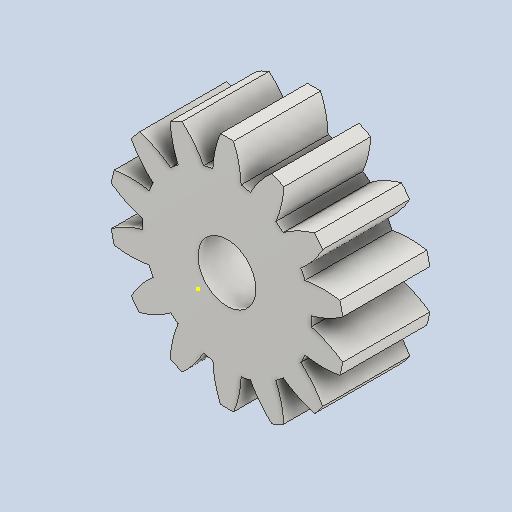
# Autodesk Inventor part: Spur Gear2
Saved by Autodesk Inventor 2022.3 (Build 263350000, 350)
## iProperties
CustomPartVersion: 1
Created: 2023-01-16
Part Number: Spur Gear2
Material: Steel
Document SubType Name: Modeling
Designer: komputer
Categories: <?xml version="1.0" encoding="UTF-16"?> <MemberInstance><Categories><FamilyTemplate><FamilyTemplateParameter ValueType="xs:double" Id="1" ObjectReferenceKey="da_z" ObjectType="kUserParameterObject"/><FamilyTemplateParameter ValueType="xs:double" Id="2" ObjectReferenceKey="da_b" ObjectType="kUserParameterObject"/><FamilyTemplateParameter ValueType="xs:double" Id="3" ObjectReferenceKey="da_beta" ObjectType="kUserParameterObject"/><FamilyTemplateParameter ValueType="xs:double" Id="4" ObjectReferenceKey="da_da" ObjectType="kUserParameterObject"/><FamilyTemplateParameter ValueType="xs:double" Id="5" ObjectReferenceKey="da_aw" ObjectType="kUserParameterObject"/><FamilyTemplateParameter ValueType="xs:string" Id="6" ObjectReferenceKey="EAIAABAAAACIAQAAAAAAAIAAAAAAAAAA" ObjectType="83910656" SubObjectId="SurfaceGeometry"/></FamilyTemplate><ParamToTemplateMap><ParamToTemplate CategoryParameter="//CategoryParameter[@InternalName='046C89C9-8512-4d59-83FE-43B91F4F132A']" TemplateParameter="1"/><ParamToTemplate CategoryParameter="//CategoryParameter[@InternalName='2552DF32-E462-4b46-AEBF-C6C7768E72AC']" TemplateParameter="2"/><ParamToTemplate CategoryParameter="//CategoryParameter[@InternalName='C9EE641D-15FC-4fae-A226-E94C4372FDD7']" TemplateParameter="3"/><ParamToTemplate><ParamToTemplate CategoryParameter="//CategoryParameter[@InternalName='00B6519A-459B-49c7-AD84-2E56D39A5744']" ConstantValue="0.000000"/></ParamToTemplate><ParamToTemplate><ParamToTemplate CategoryParameter="//CategoryParameter[@InternalName='04B31F0E-C7A6-4894-AA32-9629BEFACF47']" ConstantValue="1.000000"/></ParamToTemplate><ParamToTemplate><ParamToTemplate CategoryParameter="//CategoryParameter[@InternalName='43CBEC2E-7847-49e7-A936-2F7889FCB2D9']" ConstantValue="0.250000"/></ParamToTemplate><ParamToTemplate><ParamToTemplate CategoryParameter="//CategoryParameter[@InternalName='B1EFC894-105D-4ebd-86BF-FA20ED196853']" ConstantValue="0.350000"/></ParamToTemplate><ParamToTemplate><ParamToTemplate CategoryParameter="//CategoryParameter[@InternalName='51175063-3D10-4879-93E8-6246FE8B403D']" ConstantValue="2060000000.000000"/></ParamToTemplate><ParamToTemplate><ParamToTemplate CategoryParameter="//CategoryParameter[@InternalName='A3A52E27-4454-46a9-B0BD-C932399B70AF']" ConstantValue="0.300000"/></ParamToTemplate><ParamToTemplate><ParamToTemplate CategoryParameter="//CategoryParameter[@InternalName='91B76062-C214-41d9-B1B9-14D2AB99603D']" ConstantValue="0.050590"/></ParamToTemplate><ParamToTemplate><ParamToTemplate CategoryParameter="//CategoryParameter[@InternalName='374E806E-8B8A-4dda-A9AA-1039D6500AD2']" ConstantValue="19.766752"/></ParamToTemplate><ParamToTemplate><ParamToTemplate CategoryParameter="//CategoryParameter[@InternalName='2D373A89-B862-43d6-8D0B-0CBF12AB9F6C']" ConstantValue="0.349066"/></ParamToTemplate><ParamToTemplate CategoryParameter="//CategoryParameter[@InternalName='37777632-D6A2-4fac-9D53-DB8ACD95C989']" TemplateParameter="4"/><ParamToTemplate CategoryParameter="//CategoryParameter[@InternalName='FD1017F1-B727-4f7e-9707-0F86F1FF9423']" TemplateParameter="5"/><ParamToTemplate><ParamToTemplate CategoryParameter="//CategoryParameter[@InternalName='9E1B4470-B2D3-4ff1-B813-535BB4CDF51A']" ConstantValue="3520000.000000"/></ParamToTemplate><ParamToTemplate><ParamToTemplate CategoryParameter="//CategoryParameter[@InternalName='F8452263-BFF6-458c-9FB1-07C4B99E95CD']" ConstantValue="11400000.000000"/></ParamToTemplate><ParamToTemplate><ParamToTemplate CategoryParameter="//CategoryParameter[@InternalName='3E3BB259-FD49-497f-8171-6EBC954A3479']" ConstantValue="2.000000"/></ParamToTemplate><ParamToTemplate CategoryParameter="//CategoryParameter[@InternalName='27C3BAF2-7550-4e4b-AE2C-0DB134B7D9B7']" TemplateParameter="6"/></ParamToTemplateMap><Category DisplayName="Gear" InternalName="DC85795E-93AB-48d5-8EEE-5A27447B64BD" Mnemonic="Gear"><CategoryParameter DisplayName="z" InternalName="046C89C9-8512-4d59-83FE-43B91F4F132A" Mnemonic="z"/><CategoryParameter DisplayName="b" InternalName="2552DF32-E462-4b46-AEBF-C6C7768E72AC" Mnemonic="b"/><CategoryParameter DisplayName="||b|" InternalName="C9EE641D-15FC-4fae-A226-E94C4372FDD7" Mnemonic="beta"/><CategoryParameter DisplayName="x" InternalName="00B6519A-459B-49c7-AD84-2E56D39A5744" Mnemonic="x"/><CategoryParameter DisplayName="a*" InternalName="04B31F0E-C7A6-4894-AA32-9629BEFACF47" Mnemonic="a"/><CategoryParameter DisplayName="c*" InternalName="43CBEC2E-7847-49e7-A936-2F7889FCB2D9" Mnemonic="c"/><CategoryParameter DisplayName="r|.f|*" InternalName="B1EFC894-105D-4ebd-86BF-FA20ED196853" Mnemonic="rf"/><CategoryParameter DisplayName="E" InternalName="51175063-3D10-4879-93E8-6246FE8B403D" Mnemonic="E"/><CategoryParameter DisplayName="||m|" InternalName="A3A52E27-4454-46a9-B0BD-C932399B70AF" Mnemonic="mi"/><Category DisplayName="SpurGear" InternalName="26C5A22E-A91E-4dfd-A3B3-23CCAFAE1764" Mnemonic="SpurGear"><CategoryParameter DisplayName="m" InternalName="91B76062-C214-41d9-B1B9-14D2AB99603D" Mnemonic="m"/><CategoryParameter DisplayName="P" InternalName="374E806E-8B8A-4dda-A9AA-1039D6500AD2" Mnemonic="PP"/><CategoryParameter DisplayName="||a|" InternalName="2D373A89-B862-43d6-8D0B-0CBF12AB9F6C" Mnemonic="alpha"/><CategoryParameter DisplayName="d|.a|" InternalName="37777632-D6A2-4fac-9D53-DB8ACD95C989" Mnemonic="da"/><CategoryParameter DisplayName="a|.w|" InternalName="FD1017F1-B727-4f7e-9707-0F86F1FF9423" Mnemonic="aw"/><CategoryParameter DisplayName="||s||.Flim|" InternalName="9E1B4470-B2D3-4ff1-B813-535BB4CDF51A" Mnemonic="sFlim"/><CategoryParameter DisplayName="||s||.Hlim|" InternalName="F8452263-BFF6-458c-9FB1-07C4B99E95CD" Mnemonic="sHlim"/><CategoryParameter DisplayName="type" InternalName="3E3BB259-FD49-497f-8171-6EBC954A3479" Mnemonic="type"/><CategoryParameter DisplayName="PitchDiameter" InternalName="27C3BAF2-7550-4e4b-AE2C-0DB134B7D9B7" Mnemonic="IDS_PITCHDIAM"/></Category></Category></Categories></MemberInstance>
Density: 1 g/cm^3
Appearance: Steel
d16: 6,071 mm
d17: 0,000 mm
d41: 0,000 mm
d43: 6,071 mm
d46: 6,071 mm
d47: 0,000 mm
d48: 0,000 mm
Author: komputer
Autodesk Inventor part; units mm, degrees
sketch "Sketch1" plane through (0, 0, 0) normal (0, 0, 1) x (1, 0, 0)
  circle A0 centre (0, 0) radius 4.0472
  dimension "d0" = 8.0944
  constraints: 1 centre point
  measures "d0" diameter of A0
extrude "Extrusion1" add sketch "Sketch1" along normal blind 20
ref_plane "Work Plane2" through (0, 0, 10) normal (0, 0, 1) x (1, 0, 0)
sketch "Sketch2" plane through (0, 0, 0) normal (0, 0, -1) x (-1, 0, 0)
  circle A0 centre (0, 0) radius 4.0472 projected
  circle A1 centre (0, 0) radius 3.5413
  dimension "d3" = 7.0826
  constraints: 1 centre point, 1 coincident
  measures "d3" diameter of A1
surface extrude "Pitch Diameter" sketch "Sketch2" against normal through all shown no curves A1
ref_plane "Work Plane8" through (0, 0, 0) normal (0.9749279, 0.2225209, 0) x (0, 0, 1)
ref_plane "Work Plane9" through (0, 0, 0) normal (1, 0, 0) x (0, 1, 0)
spur gear teeth "Spur Gear" teeth 14 pitch diameter 7.0826 tip diameter 8.0944 root diameter 5.8178 face width 20 start plane through (0, 0, 0) normal (0, 0, -1) x (-1, 0, 0)
sketch "Sketch3" plane through (0, 0, 20) normal (0, 0, 1) x (1, 0, 0)
  arc A0 (-1.9577, 3.5422) -> (-1.6833, 2.3724) centre (1.4737, 3.73) ccw projected
  arc A1 (-1.6833, 2.3724) -> (-1.9384, 2.169) centre (0, 0) ccw projected
  arc A2 (-1.9384, 2.169) -> (-3.0178, 2.6968) centre (-3.9644, -0.6067) ccw projected
  arc A3 (-3.0178, 2.6968) -> (-3.3007, 2.342) centre (0, 0) ccw projected
  arc A4 (-3.3007, 2.342) -> (-2.546, 1.4071) centre (-0.2907, 4) ccw projected
  arc A5 (-2.546, 1.4071) -> (-2.6875, 1.1132) centre (0, 0) ccw projected
  arc A6 (-2.6875, 1.1132) -> (-3.889, 1.1204) centre (-3.3086, -2.2667) ccw projected
  arc A7 (-3.889, 1.1204) -> (-3.99, 0.6779) centre (0, 0) ccw projected
  arc A8 (-3.99, 0.6779) -> (-2.9043, 0.1631) centre (-1.9974, 3.4778) ccw projected
  arc A9 (-2.9043, 0.1631) -> (-2.9043, -0.1631) centre (0, 0) ccw projected
  arc A10 (-2.9043, -0.1631) -> (-3.99, -0.6779) centre (-1.9974, -3.4778) ccw projected
  arc A11 (-3.99, -0.6779) -> (-3.889, -1.1204) centre (0, 0) ccw projected
  arc A12 (-3.889, -1.1204) -> (-2.6875, -1.1132) centre (-3.3086, 2.2667) ccw projected
  arc A13 (-2.6875, -1.1132) -> (-2.546, -1.4071) centre (0, 0) ccw projected
  arc A14 (-2.546, -1.4071) -> (-3.3007, -2.342) centre (-0.2907, -4) ccw projected
  arc A15 (-3.3007, -2.342) -> (-3.0178, -2.6968) centre (0, 0) ccw projected
  arc A16 (-3.0178, -2.6968) -> (-1.9384, -2.169) centre (-3.9644, 0.6067) ccw projected
  arc A17 (-1.9384, -2.169) -> (-1.6833, -2.3724) centre (0, 0) ccw projected
  arc A18 (-1.6833, -2.3724) -> (-1.9577, -3.5422) centre (1.4737, -3.73) ccw projected
  arc A19 (-1.9577, -3.5422) -> (-1.5488, -3.7391) centre (0, 0) ccw projected
  arc A20 (-1.5488, -3.7391) -> (-0.8053, -2.7952) centre (-3.8351, -1.1735) ccw projected
  arc A21 (-0.8053, -2.7952) -> (-0.4873, -2.8678) centre (0, 0) ccw projected
  arc A22 (-0.4873, -2.8678) -> (-0.2269, -4.0408) centre (2.9461, -2.7212) ccw projected
  arc A23 (-0.2269, -4.0408) -> (0.2269, -4.0408) centre (0, 0) ccw projected
  arc A24 (0.2269, -4.0408) -> (0.4873, -2.8678) centre (-2.9461, -2.7212) ccw projected
  arc A25 (0.4873, -2.8678) -> (0.8053, -2.7952) centre (0, 0) ccw projected
  arc A26 (0.8053, -2.7952) -> (1.5488, -3.7391) centre (3.8351, -1.1735) ccw projected
  arc A27 (1.5488, -3.7391) -> (1.9577, -3.5422) centre (0, 0) ccw projected
  arc A28 (1.9577, -3.5422) -> (1.6833, -2.3724) centre (-1.4737, -3.73) ccw projected
  arc A29 (1.6833, -2.3724) -> (1.9384, -2.169) centre (0, 0) ccw projected
  arc A30 (1.9384, -2.169) -> (3.0178, -2.6968) centre (3.9644, 0.6067) ccw projected
  arc A31 (3.0178, -2.6968) -> (3.3007, -2.342) centre (0, 0) ccw projected
  arc A32 (3.3007, -2.342) -> (2.546, -1.4071) centre (0.2907, -4) ccw projected
  arc A33 (2.546, -1.4071) -> (2.6875, -1.1132) centre (0, 0) ccw projected
  arc A34 (2.6875, -1.1132) -> (3.889, -1.1204) centre (3.3086, 2.2667) ccw projected
  arc A35 (3.889, -1.1204) -> (3.99, -0.6779) centre (0, 0) ccw projected
  arc A36 (3.99, -0.6779) -> (2.9043, -0.1631) centre (1.9974, -3.4778) ccw projected
  arc A37 (2.9043, -0.1631) -> (2.9043, 0.1631) centre (0, 0) ccw projected
  arc A38 (2.9043, 0.1631) -> (3.99, 0.6779) centre (1.9974, 3.4778) ccw projected
  arc A39 (3.99, 0.6779) -> (3.889, 1.1204) centre (0, 0) ccw projected
  arc A40 (3.889, 1.1204) -> (2.6875, 1.1132) centre (3.3086, -2.2667) ccw projected
  arc A41 (2.6875, 1.1132) -> (2.546, 1.4071) centre (0, 0) ccw projected
  arc A42 (2.546, 1.4071) -> (3.3007, 2.342) centre (0.2907, 4) ccw projected
  arc A43 (3.3007, 2.342) -> (3.0178, 2.6968) centre (0, 0) ccw projected
  arc A44 (3.0178, 2.6968) -> (1.9384, 2.169) centre (3.9644, -0.6067) ccw projected
  arc A45 (1.9384, 2.169) -> (1.6833, 2.3724) centre (0, 0) ccw projected
  arc A46 (1.6833, 2.3724) -> (1.9577, 3.5422) centre (-1.4737, 3.73) ccw projected
  arc A47 (1.9577, 3.5422) -> (1.5488, 3.7391) centre (0, 0) ccw projected
  arc A48 (1.5488, 3.7391) -> (0.8053, 2.7952) centre (3.8351, 1.1735) ccw projected
  arc A49 (0.8053, 2.7952) -> (0.4873, 2.8678) centre (0, 0) ccw projected
  arc A50 (0.4873, 2.8678) -> (0.2269, 4.0408) centre (-2.9461, 2.7212) ccw projected
  arc A51 (0.2269, 4.0408) -> (-0.2269, 4.0408) centre (0, 0) ccw projected
  arc A52 (-0.2269, 4.0408) -> (-0.4873, 2.8678) centre (2.9461, 2.7212) ccw projected
  arc A53 (-0.4873, 2.8678) -> (-0.8053, 2.7952) centre (0, 0) ccw projected
  arc A54 (-0.8053, 2.7952) -> (-1.5488, 3.7391) centre (-3.8351, 1.1735) ccw projected
  arc A55 (-1.5488, 3.7391) -> (-1.9577, 3.5422) centre (0, 0) ccw projected
  arc A56 (3.889, -1.1204) -> (3.99, -0.6779) centre (0, 0) ccw projected
  arc A57 (3.0178, -2.6968) -> (3.3007, -2.342) centre (0, 0) ccw projected
  line L0 (3.889, -1.1204) -> (3.3007, -2.342)
  line L1 (-3.889, 1.1204) -> (-3.3007, 2.342)
  arc A58 (-3.0178, 2.6968) -> (-3.3007, 2.342) centre (0, 0) ccw projected
  circle A59 centre (0, 0) radius 1
  dimension "d49" = 2
  constraints: 4 end point, 1 centre point, 1 coincident, 1 point on circle
  measures "d49" diameter of A59
extrude "Extrusion2" cut sketch "Sketch3" against normal blind 16 contours A55 A54 A53 A52 A51 A50 A49 A48 A47 A46 A45 A44 A43 A42 A41 A40 A39 A38 A37 A36 A35 A34 A33 A32 A31 A30 A29 A28 A27 A26 A25 A24 A23 A22 A21 A20 A19 A18 A17 A16 A15 A14 A13 A12 A11 A10 A9 A8 A7 A6 A5 A4 A3 A2 A1 A0 | A59
extrude "Extrusion3" cut sketch "Sketch3" against normal through all contours A59
sketch "Sketch4" plane through (0, 0, 4) normal (0, 0, 1) x (1, 0, 0)
  point P0 (0, 0)
sketch "Sketch5" plane through (0, 0, 4) normal (0, 0, 1) x (1, 0, 0)
  circle A0 centre (0, 0) radius 1 projected
  arc A1 (-3.0178, 2.6968) -> (-3.3007, 2.342) centre (0, 0) ccw projected
  arc A2 (-3.3007, 2.342) -> (-2.546, 1.4071) centre (-0.2907, 4) ccw projected
  arc A3 (-2.546, 1.4071) -> (-2.6875, 1.1132) centre (0, 0) ccw projected
  arc A4 (-2.6875, 1.1132) -> (-3.889, 1.1204) centre (-3.3086, -2.2667) ccw projected
  arc A5 (-3.889, 1.1204) -> (-3.99, 0.6779) centre (0, 0) ccw projected
  arc A6 (-3.99, 0.6779) -> (-2.9043, 0.1631) centre (-1.9974, 3.4778) ccw projected
  arc A7 (-2.9043, 0.1631) -> (-2.9043, -0.1631) centre (0, 0) ccw projected
  arc A8 (-2.9043, -0.1631) -> (-3.99, -0.6779) centre (-1.9974, -3.4778) ccw projected
  arc A9 (-3.99, -0.6779) -> (-3.889, -1.1204) centre (0, 0) ccw projected
  arc A10 (-3.889, -1.1204) -> (-2.6875, -1.1132) centre (-3.3086, 2.2667) ccw projected
  arc A11 (-2.6875, -1.1132) -> (-2.546, -1.4071) centre (0, 0) ccw projected
  arc A12 (-2.546, -1.4071) -> (-3.3007, -2.342) centre (-0.2907, -4) ccw projected
  arc A13 (-3.3007, -2.342) -> (-3.0178, -2.6968) centre (0, 0) ccw projected
  arc A14 (-3.0178, -2.6968) -> (-1.9384, -2.169) centre (-3.9644, 0.6067) ccw projected
  arc A15 (-1.9384, -2.169) -> (-1.6833, -2.3724) centre (0, 0) ccw projected
  arc A16 (-1.6833, -2.3724) -> (-1.9577, -3.5422) centre (1.4737, -3.73) ccw projected
  arc A17 (-1.9577, -3.5422) -> (-1.5488, -3.7391) centre (0, 0) ccw projected
  arc A18 (-1.5488, -3.7391) -> (-0.8053, -2.7952) centre (-3.8351, -1.1735) ccw projected
  arc A19 (-0.8053, -2.7952) -> (-0.4873, -2.8678) centre (0, 0) ccw projected
  arc A20 (-0.4873, -2.8678) -> (-0.2269, -4.0408) centre (2.9461, -2.7212) ccw projected
  arc A21 (-0.2269, -4.0408) -> (0.2269, -4.0408) centre (0, 0) ccw projected
  arc A22 (0.2269, -4.0408) -> (0.4873, -2.8678) centre (-2.9461, -2.7212) ccw projected
  arc A23 (0.4873, -2.8678) -> (0.8053, -2.7952) centre (0, 0) ccw projected
  arc A24 (0.8053, -2.7952) -> (1.5488, -3.7391) centre (3.8351, -1.1735) ccw projected
  arc A25 (1.5488, -3.7391) -> (1.9577, -3.5422) centre (0, 0) ccw projected
  arc A26 (1.9577, -3.5422) -> (1.6833, -2.3724) centre (-1.4737, -3.73) ccw projected
  arc A27 (1.6833, -2.3724) -> (1.9384, -2.169) centre (0, 0) ccw projected
  arc A28 (1.9384, -2.169) -> (3.0178, -2.6968) centre (3.9644, 0.6067) ccw projected
  arc A29 (3.0178, -2.6968) -> (3.3007, -2.342) centre (0, 0) ccw projected
  arc A30 (3.3007, -2.342) -> (2.546, -1.4071) centre (0.2907, -4) ccw projected
  arc A31 (2.546, -1.4071) -> (2.6875, -1.1132) centre (0, 0) ccw projected
  arc A32 (2.6875, -1.1132) -> (3.889, -1.1204) centre (3.3086, 2.2667) ccw projected
  arc A33 (3.889, -1.1204) -> (3.99, -0.6779) centre (0, 0) ccw projected
  arc A34 (3.99, -0.6779) -> (2.9043, -0.1631) centre (1.9974, -3.4778) ccw projected
  arc A35 (2.9043, -0.1631) -> (2.9043, 0.1631) centre (0, 0) ccw projected
  arc A36 (2.9043, 0.1631) -> (3.99, 0.6779) centre (1.9974, 3.4778) ccw projected
  arc A37 (3.99, 0.6779) -> (3.889, 1.1204) centre (0, 0) ccw projected
  arc A38 (3.889, 1.1204) -> (2.6875, 1.1132) centre (3.3086, -2.2667) ccw projected
  arc A39 (2.6875, 1.1132) -> (2.546, 1.4071) centre (0, 0) ccw projected
  arc A40 (2.546, 1.4071) -> (3.3007, 2.342) centre (0.2907, 4) ccw projected
  arc A41 (3.3007, 2.342) -> (3.0178, 2.6968) centre (0, 0) ccw projected
  arc A42 (3.0178, 2.6968) -> (1.9384, 2.169) centre (3.9644, -0.6067) ccw projected
  arc A43 (1.9384, 2.169) -> (1.6833, 2.3724) centre (0, 0) ccw projected
  arc A44 (1.6833, 2.3724) -> (1.9577, 3.5422) centre (-1.4737, 3.73) ccw projected
  arc A45 (1.9577, 3.5422) -> (1.5488, 3.7391) centre (0, 0) ccw projected
  arc A46 (1.5488, 3.7391) -> (0.8053, 2.7952) centre (3.8351, 1.1735) ccw projected
  arc A47 (0.8053, 2.7952) -> (0.4873, 2.8678) centre (0, 0) ccw projected
  arc A48 (0.4873, 2.8678) -> (0.2269, 4.0408) centre (-2.9461, 2.7212) ccw projected
  arc A49 (0.2269, 4.0408) -> (-0.2269, 4.0408) centre (0, 0) ccw projected
  arc A50 (-0.2269, 4.0408) -> (-0.4873, 2.8678) centre (2.9461, 2.7212) ccw projected
  arc A51 (-0.4873, 2.8678) -> (-0.8053, 2.7952) centre (0, 0) ccw projected
  arc A52 (-0.8053, 2.7952) -> (-1.5488, 3.7391) centre (-3.8351, 1.1735) ccw projected
  arc A53 (-1.5488, 3.7391) -> (-1.9577, 3.5422) centre (0, 0) ccw projected
  arc A54 (-1.9577, 3.5422) -> (-1.6833, 2.3724) centre (1.4737, 3.73) ccw projected
  arc A55 (-1.6833, 2.3724) -> (-1.9384, 2.169) centre (0, 0) ccw projected
  arc A56 (-1.9384, 2.169) -> (-3.0178, 2.6968) centre (-3.9644, -0.6067) ccw projected
extrude "Extrusion4" cut sketch "Sketch5" against normal blind 1
equation "\"d0\" = da_da"
equation "\"d1\" = da_b"
equation "\"d3\" = da_d"
equation "\"d16\" = da_aw"
equation "\"d43\" = da_aw"
equation "\"d46\" = da_aw"
equation "\"da_da\" = 8.0944"
equation "\"da_b\" = 20"
equation "\"da_d\" = 7.0826"
equation "\"da_aw\" = 6.0708"
body "Solid1"
body "Srf1"
